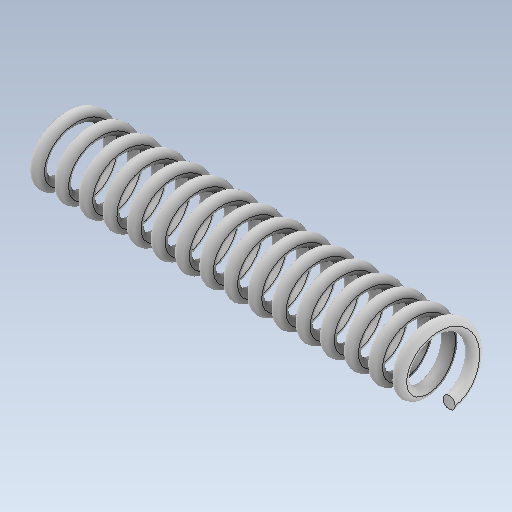
# Autodesk Inventor part: Part6
Saved by Autodesk Inventor 2021 (Build 250183000, 183)
## iProperties
Created: 2022-06-05
Part Number: Part6
Material: Generic
Document SubType Name: Modeling
Designer: Bhargav Malasani
Density: 1 g/cm^3
Appearance: Default
Author: Bhargav Malasani
Autodesk Inventor part; units mm, degrees
ref_plane "YZ Plane" through (0, 0, 0) normal (1, 0, 0) x (0, 1, 0)
ref_plane "XZ Plane" through (0, 0, 0) normal (0, 1, 0) x (-1, 0, 0)
ref_plane "XY Plane" through (0, 0, 0) normal (0, 0, 1) x (1, 0, 0)
sketch "Sketch1" plane through (0, 0, 0) normal (0, 0, 1) x (1, 0, 0)
  line L0 (0, 0) -> (198, 0)
  circle A0 centre (198, -15) radius 3
  circle A1 centre (186, -15) radius 3
  dimension "d0" = 198
  dimension "d1" = 6
  dimension "d2" = 6
  dimension "d3" = 15
  dimension "d4" = 15
  dimension "d5" = 198
  dimension "d6" = 12
  constraints: 2 centre point, 2 end point, 1 horizontal
  measures "d0" distance of L0.start L0.end
  measures "d1" diameter of A0
  measures "d2" diameter of A1
  measures "d3" distance from line of L0 A0.centre
  measures "d4" distance from line of L0 A1.centre
  measures "d5" horizontal distance of L0.start A0.centre
  measures "d6" distance of A1.centre A0.centre
coil "Coil1" sketch "Sketch1" operation add axis through (0, 0, 0) along (-1, 0, 0) pitch 12 turns 16 hand left contours A1
equation "\"d4\" = d3"
body "Solid1"
